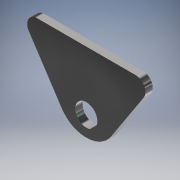
# Autodesk Inventor part: bearingplaterear
Saved by Autodesk Inventor 2018 (Build 220112000, 112)
## iProperties
Created: 2018-07-30
Part Number: bearingplaterear
Material: Steel, Mild
Document SubType Name: Modeling
Designer: Cole Tucker
Density: 7.85 g/cm^3
Appearance: Semi-Polished
Mass: 729.659 g
Surface Area: 243.887 cm^2
Volume: 92.9502 cm^3
Author: Cole Tucker
Autodesk Inventor part; units mm, degrees
ref_plane "YZ Plane" through (0, 0, 0) normal (1, 0, 0) x (0, 1, 0)
ref_plane "XZ Plane" through (0, 0, 0) normal (0, 1, 0) x (-1, 0, 0)
ref_plane "XY Plane" through (0, 0, 0) normal (0, 0, 1) x (1, 0, 0)
sketch "Sketch1" plane through (0, 0, 0) normal (0, 0, 1) x (1, 0, 0)
  circle A0 centre (-12.7, 12.7) radius 38.1
  line L0 (-12.7, 12.7) -> (-12.7, 63.5)
  line L1 (-12.7, 63.5) -> (50.8, 63.5)
  line L2 (-12.7, 63.5) -> (-76.2, 63.5)
  circle A1 centre (-76.2, 63.5) radius 12.7
  circle A2 centre (50.8, 63.5) radius 12.7
  line L3 (-76.2, 76.2) -> (50.8, 76.2)
  line L4 (-86.8343, 56.5572) -> (-44.6028, -8.1284)
  line L5 (61.4343, 56.5572) -> (19.2028, -8.1284)
  point P0 (0, 0)
  dimension "d1" = 76.2
  dimension "d2" = 50.8
  dimension "d3" = 63.5
  dimension "d4" = 63.5
  dimension "d5" = 25.4
  dimension "d6" = 25.4
  constraints: 12 end point, 6 point on circle, 5 coincident, 5 tangent, 3 centre point, 2 horizontal, 1 perpendicular, 1 vertical
  measures "d1" diameter of A0
  measures "d2" distance of L0.start L0.end
  measures "d3" distance of L0.end L1.end
  measures "d4" distance of L0.end L2.end
  measures "d5" diameter of A1
  measures "d6" diameter of A2
extrude "Extrusion2" add sketch "Sketch1" along normal blind 9.525
sketch "Sketch3" plane through (0, 0, 9.525) normal (0, 0, 1) x (1, 0, 0)
  line L0 (50.8, 76.2) -> (-76.2, 76.2) construction
  line L1 (-12.7, 76.2) -> (-12.7, -25.4) construction
  arc A0 (-44.6028, -8.1284) -> (19.2028, -8.1284) centre (-12.7, 12.7) ccw construction
  point P0 (0, 0)
  point P1 (-12.7, 0)
  dimension "d40" = 25.4
  constraints: 2 end point, 1 midpoint, 1 point on circle, 1 point on line, 1 vertical
  measures "d40" distance of L1.end point (-12.7, 0)
hole "Hole4" at (-12.7, 0, 9.525) direction (0, 0, -1) diameter 28.575 depth 25.4 tip angle 118
equation "\"d3\" = d4"
body "Solid2"
